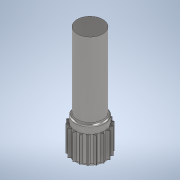
# Autodesk Inventor part: Wałek_Sprzęgłowy
Saved by Autodesk Inventor 2022 (Build 260153000, 153)
## iProperties
Created: 2021-11-28
Part Number: Wałek_Sprzęgłowy
Material: Stal, stopowa
Document SubType Name: Modeling
Designer: Mateu
Density: 7.73 g/cm^3
Appearance: Częściowo polerowany
Author: Mateu
Autodesk Inventor part; units mm, degrees
ref_plane "YZ Plane" through (0, 0, 0) normal (1, 0, 0) x (0, 1, 0)
ref_plane "XZ Plane" through (0, 0, 0) normal (0, 1, 0) x (-1, 0, 0)
ref_plane "XY Plane" through (0, 0, 0) normal (0, 0, 1) x (1, 0, 0)
sketch "Szkic1" plane through (0, 0, 0) normal (0, 1, 0) x (-1, 0, 0)
  circle A0 centre (0, 0) radius 13.5
  line L0 (13.5, 0) -> (11.5, 0)
  line L1 (11.5, 0) -> (11.5, -1)
  line L2 (11.5, 0) -> (11.5, 1)
  line L3 (11.5, -1) -> (13.3084, -2.2663)
  line L4 (11.5, -1) -> (13.7077, -1) construction
  line L5 (11.5, 1) -> (13.3084, 2.2663)
  line L6 (10.4644, 4.8729) -> (11.7307, 6.6813)
  line L7 (10.8065, 3.9332) -> (10.4644, 4.8729)
  line L8 (10.8065, 3.9332) -> (11.1485, 2.9935)
  line L9 (11.1485, 2.9935) -> (13.2809, 2.4222)
  line L10 (8.1667, 8.1581) -> (8.7381, 10.2905)
  line L11 (8.8095, 7.3921) -> (8.1667, 8.1581)
  line L12 (8.8095, 7.3921) -> (9.4523, 6.626)
  line L13 (9.4523, 6.626) -> (11.6516, 6.8184)
  line L14 (4.884, 10.4593) -> (4.6916, 12.6586)
  line L15 (5.75, 9.9593) -> (4.884, 10.4593)
  line L16 (5.75, 9.9593) -> (6.616, 9.4593)
  line L17 (6.616, 9.4593) -> (8.6169, 10.3923)
  line L18 (1.0121, 11.4989) -> (0.0791, 13.4998)
  line L19 (1.997, 11.3253) -> (1.0121, 11.4989)
  line L20 (1.997, 11.3253) -> (2.9818, 11.1516)
  line L21 (2.9818, 11.1516) -> (4.5428, 12.7127)
  line L22 (-2.9818, 11.1516) -> (-4.5428, 12.7127)
  line L23 (-1.997, 11.3253) -> (-2.9818, 11.1516)
  line L24 (-1.997, 11.3253) -> (-1.0121, 11.4989)
  line L25 (-1.0121, 11.4989) -> (-0.0791, 13.4998)
  line L26 (-6.616, 9.4593) -> (-8.6169, 10.3923)
  line L27 (-5.75, 9.9593) -> (-6.616, 9.4593)
  line L28 (-5.75, 9.9593) -> (-4.884, 10.4593)
  line L29 (-4.884, 10.4593) -> (-4.6916, 12.6586)
  line L30 (-9.4523, 6.626) -> (-11.6516, 6.8184)
  line L31 (-8.8095, 7.3921) -> (-9.4523, 6.626)
  line L32 (-8.8095, 7.3921) -> (-8.1667, 8.1581)
  line L33 (-8.1667, 8.1581) -> (-8.7381, 10.2905)
  line L34 (-11.1485, 2.9935) -> (-13.2809, 2.4222)
  line L35 (-10.8065, 3.9332) -> (-11.1485, 2.9935)
  line L36 (-10.8065, 3.9332) -> (-10.4644, 4.8729)
  line L37 (-10.4644, 4.8729) -> (-11.7307, 6.6813)
  line L38 (-11.5, -1) -> (-13.3084, -2.2663)
  line L39 (-11.5, 0) -> (-11.5, -1)
  line L40 (-11.5, 0) -> (-11.5, 1)
  line L41 (-11.5, 1) -> (-13.3084, 2.2663)
  line L42 (-10.4644, -4.8729) -> (-11.7307, -6.6813)
  line L43 (-10.8065, -3.9332) -> (-10.4644, -4.8729)
  line L44 (-10.8065, -3.9332) -> (-11.1485, -2.9935)
  line L45 (-11.1485, -2.9935) -> (-13.2809, -2.4222)
  line L46 (-8.1667, -8.1581) -> (-8.7381, -10.2905)
  line L47 (-8.8095, -7.3921) -> (-8.1667, -8.1581)
  line L48 (-8.8095, -7.3921) -> (-9.4523, -6.626)
  line L49 (-9.4523, -6.626) -> (-11.6516, -6.8184)
  line L50 (-4.884, -10.4593) -> (-4.6916, -12.6586)
  line L51 (-5.75, -9.9593) -> (-4.884, -10.4593)
  line L52 (-5.75, -9.9593) -> (-6.616, -9.4593)
  line L53 (-6.616, -9.4593) -> (-8.6169, -10.3923)
  line L54 (-1.0121, -11.4989) -> (-0.0791, -13.4998)
  line L55 (-1.997, -11.3253) -> (-1.0121, -11.4989)
  line L56 (-1.997, -11.3253) -> (-2.9818, -11.1516)
  line L57 (-2.9818, -11.1516) -> (-4.5428, -12.7127)
  line L58 (2.9818, -11.1516) -> (4.5428, -12.7127)
  line L59 (1.997, -11.3253) -> (2.9818, -11.1516)
  line L60 (1.997, -11.3253) -> (1.0121, -11.4989)
  line L61 (1.0121, -11.4989) -> (0.0791, -13.4998)
  line L62 (6.616, -9.4593) -> (8.6169, -10.3923)
  line L63 (5.75, -9.9593) -> (6.616, -9.4593)
  line L64 (5.75, -9.9593) -> (4.884, -10.4593)
  line L65 (4.884, -10.4593) -> (4.6916, -12.6586)
  line L66 (9.4523, -6.626) -> (11.6516, -6.8184)
  line L67 (8.8095, -7.3921) -> (9.4523, -6.626)
  line L68 (8.8095, -7.3921) -> (8.1667, -8.1581)
  line L69 (8.1667, -8.1581) -> (8.7381, -10.2905)
  line L70 (11.1485, -2.9935) -> (13.2809, -2.4222)
  line L71 (10.8065, -3.9332) -> (11.1485, -2.9935)
  line L72 (10.8065, -3.9332) -> (10.4644, -4.8729)
  line L73 (10.4644, -4.8729) -> (11.7307, -6.6813)
  dimension "d0" = 27
  dimension "d2" = 1
  dimension "d3" = 1
  dimension "d5" = 35
  dimension "d8" = 360
  constraints: 148 end point, 2 horizontal, 2 vertical, 1 coincident, 1 equal length, 1 symmetric about line, 167 other
  measures "d2" distance of L0.end L1.end
  measures "d3" distance of L0.end L2.end
  measures "d5" angle of L3 L4
extrude "Wyciągnięcie proste1" add sketch "Szkic1" along normal blind 20 contours L5 L2 L1 L3 A0 L70 L71 L72 L73 L66 L67 L68 L69 L62 L63 L64 L65 L58 L59 L60 L61 L54 L55 L56 L57 L50 L51 L52 L53 L46 L47 L48 L49 L42 L43 L44 L45 L38 L39 L40 L41 L34 L35 L36 L37 L30 L31 L32 L33 L26 L27 L28 L29 L22 L23 L24 L25 L18 L19 L20 L21 L14 L15 L16 L17 L10 L11 L12 L13 L6 L7 L8 L9
sketch "Szkic2" plane through (0, 20, 0) normal (0, 1, 0) x (1, 0, 0)
  circle A0 centre (0, 0) radius 11.5
  constraints: 1 centre point, 1 coincident
extrude "Wyciągnięcie proste2" add sketch "Szkic2" along normal blind 5
sketch "Szkic3" plane through (0, 25, 0) normal (0, 1, 0) x (1, 0, 0)
  circle A0 centre (0, 0) radius 10
  dimension "d15" = 20
  constraints: 1 centre point, 1 coincident
  measures "d15" diameter of A0
extrude "Wyciągnięcie proste3" add sketch "Szkic3" along normal blind 60
fillet "Zaokrąglenie1" radius 2 1 edges at (-10, 25, 0)
sketch "Szkic4" plane through (0, 0, 0) normal (0, -1, 0) x (1, 0, 0)
  arc A0 (5.75, 9.9593) -> (1.997, 11.3253) centre (0, 0) ccw projected
  circle A1 centre (0, 0) radius 11.5
  point P0 (5.75, 9.9593)
  constraints: 1 coincident, 3 other
extrude "Wyciągnięcie proste4" add sketch "Szkic4" along normal blind 1
